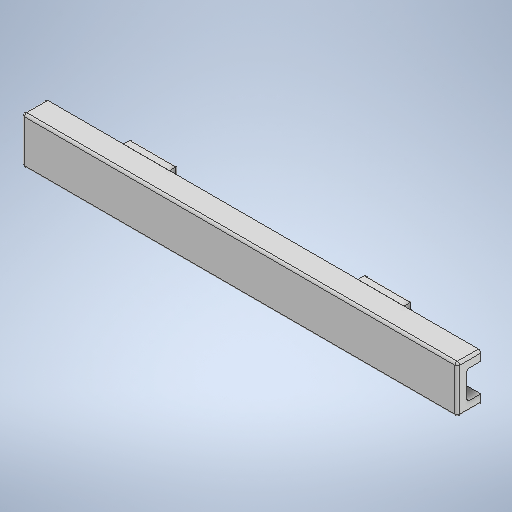
# Autodesk Inventor part: Kabelschacht 001
Saved by Autodesk Inventor 2025 (Build 290162000, 162)
## iProperties
Created: 2024-04-08
Part Number: Kabelschacht 001
Material: Generisch
Document SubType Name: Modeling
Designer: noahm
Density: 1 g/cm^3
Appearance: Vorgabe
Author: noahm
Autodesk Inventor part; units mm, degrees
ref_plane "YZ Plane" through (0, 0, 0) normal (1, 0, 0) x (0, 1, 0)
ref_plane "XZ Plane" through (0, 0, 0) normal (0, 1, 0) x (-1, 0, 0)
ref_plane "XY Plane" through (0, 0, 0) normal (0, 0, 1) x (1, 0, 0)
sketch "Skizze1" plane through (0, 0, 0) normal (0, 1, 0) x (-1, 0, 0)
  line L0 (-92.5, -10) -> (92.5, -10)
  line L1 (92.5, -10) -> (92.5, 10)
  line L2 (92.5, 10) -> (-92.5, 10)
  line L3 (-92.5, 10) -> (-92.5, -10)
  line L4 (-92.5, -10) -> (92.5, 10) construction
  line L5 (92.5, -10) -> (-92.5, 10) construction
  point P0 (0, 0)
  dimension "d0" = 20
  dimension "d1" = 185
  constraints: 12 end point, 2 midpoint, 2 parallel, 1 horizontal, 1 perpendicular
  measures "d0" distance of L0.end L1.end
  measures "d1" distance of L1.end L2.end
extrude "Extrusion1" add sketch "Skizze1" along normal blind 10
sketch "Skizze2" plane through (92.5, 0, 10) normal (1, 0, 0) x (0, 0, -1)
  line L0 (20, 10) -> (0, 10) projected
  line L1 (4, 10) -> (16, 10)
  line L2 (16, 10) -> (16, 4)
  line L3 (16, 4) -> (4, 4)
  line L4 (4, 4) -> (4, 10)
  line L5 (0, 0) -> (0, 10) projected
  line L6 (20, 0) -> (20, 10) projected
  line L7 (0, 0) -> (20, 0) projected
  point P0 (10, 0)
  point P1 (16, 7)
  point P2 (10, 4)
  dimension "d4" = 4
  dimension "d5" = 4
  dimension "d6" = 4
  constraints: 8 end point, 2 midpoint, 2 parallel, 1 horizontal, 1 perpendicular, 1 point on line
  measures "d4" distance between parallel lines of L5 L4
  measures "d5" distance from line of L6 point (16, 7)
  measures "d6" distance from line of L7 point (10, 4)
extrude "Extrusion2" cut sketch "Skizze2" against normal blind 181 contours L2 L3 L4 L0
sketch "Skizze3" plane through (0, 10, 0) normal (0, 1, 0) x (1, 0, 0)
  line L0 (-59.65, -9.75) -> (-40.05, -9.75)
  line L1 (-40.05, -9.75) -> (-40.05, -6.25)
  line L2 (-40.05, -6.25) -> (-59.65, -6.25)
  line L3 (-59.65, -6.25) -> (-59.65, -9.75)
  line L4 (-92.5, 10) -> (-92.5, -10) projected
  line L5 (92.5, -6) -> (-88.5, -6) projected
  line L6 (-59.65, 6.25) -> (-40, 6.25)
  line L7 (-40, 6.25) -> (-40, 9.75)
  line L8 (-40, 9.75) -> (-59.65, 9.75)
  line L9 (-59.65, 9.75) -> (-59.65, 6.25)
  line L10 (-88.5, 6) -> (92.5, 6) projected
  line L11 (40.05, -9.75) -> (59.65, -9.75)
  line L12 (59.65, -9.75) -> (59.65, -6.25)
  line L13 (59.65, -6.25) -> (40.05, -6.25)
  line L14 (40.05, -6.25) -> (40.05, -9.75)
  line L15 (92.5, -10) -> (92.5, -6) projected
  line L16 (40.0125, 6.25) -> (59.65, 6.25)
  line L17 (59.65, 6.25) -> (59.65, 9.75)
  line L18 (59.65, 9.75) -> (40.0125, 9.75)
  line L19 (40.0125, 9.75) -> (40.0125, 6.25)
  point P0 (0, 0)
  point P1 (-59.65, -8)
  point P2 (92.5, -8)
  point P3 (59.65, -8)
  dimension "d9" = 3.5
  dimension "d10" = 32.85
  dimension "d11" = 0.25
  dimension "d12" = 19.6
  dimension "d13" = 0.25
  dimension "d14" = 3.5
  dimension "d15" = 32.85
  dimension "d16" = 0.25
  dimension "d17" = 19.6
  dimension "d18" = 3.5
  dimension "d19" = 0.25
  dimension "d20" = 3.5
  dimension "d23" = 0
  dimension "d24" = 0
  constraints: 32 end point, 8 parallel, 4 horizontal, 4 perpendicular, 3 midpoint
  measures "d9" distance of L2.end L0.start
  measures "d10" distance from line of L4 point (-59.65, -8)
  measures "d11" distance between parallel lines of L5 L2
  measures "d12" distance of L1.end L2.end
  measures "d13" distance between parallel lines of L10 L6
  measures "d14" distance of L8.end L6.start
  measures "d15" distance of point (92.5, -8) point (59.65, -8)
  measures "d16" distance between parallel lines of L5 L13
  measures "d17" distance of L11.start L11.end
  measures "d18" distance of L13.end L11.start
  measures "d19" distance between parallel lines of L10 L16
  measures "d20" distance of L18.end L16.start
  measures "d23" distance between parallel lines of L17 L12
  measures "d24" distance between parallel lines of L3 L9
extrude "Extrusion3" add sketch "Skizze3" along normal blind 3.925
fillet "Rundung1" radius 1 26 edges at (-49.85, 13.925, 9.75) (-49.85, 13.925, 6.25) (-59.65, 13.925, 8) (-40.05, 13.925, 8) (-59.65, 13.925, -8) (-49.825, 13.925, -6.25) (-49.825, 13.925, -9.75) (-40, 13.925, -8) (40.0125, 13.925, -8) (49.8312, 13.925, -9.75) (49.8312, 13.925, -6.25) (59.65, 13.925, -8) (40.05, 13.925, 8) (49.85, 13.925, 9.75) (49.85, 13.925, 6.25) (59.65, 13.925, 8) (92.5, 5, 10) (92.5, 5, -10) (-92.5, 5, -10) (-92.5, 5, 10) (-92.5, 0, 0) (0, 0, 10) (0, 0, -10) (92.5, 0, 0) (2, 4, -6) (2, 4, 6)
